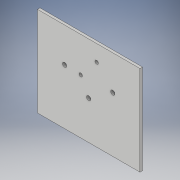
# Autodesk Inventor part: 板
Saved by Autodesk Inventor 2019 (Build 230136000, 136)
## iProperties
Created: 2020-09-25
Part Number: 板
Material: 一般
Document SubType Name: Modeling
Designer: Toshihito
Density: 1 g/cm^3
Appearance: 既定
Author: Toshihito
Autodesk Inventor part; units mm, degrees
ref_plane "YZ Plane" through (0, 0, 0) normal (1, 0, 0) x (0, 1, 0)
ref_plane "XZ Plane" through (0, 0, 0) normal (0, 1, 0) x (-1, 0, 0)
ref_plane "XY Plane" through (0, 0, 0) normal (0, 0, 1) x (1, 0, 0)
sketch "スケッチ1" plane through (0, 0, 0) normal (0, 0, 1) x (1, 0, 0)
  line L0 (-60, 52.5) -> (60, 52.5)
  line L1 (60, 52.5) -> (60, -52.5)
  line L2 (60, -52.5) -> (-60, -52.5)
  line L3 (-60, -52.5) -> (-60, 52.5)
  line L4 (-60, 52.5) -> (60, -52.5) construction
  line L5 (60, 52.5) -> (-60, -52.5) construction
  line L6 (-105.2334, 22.5) -> (96.2645, 22.5) construction
  circle A0 centre (0, -7.5) radius 2.5
  line L7 (0, 22.5) -> (28.1908, 12.2394) construction
  line L8 (0, 22.5) -> (-28.1908, 12.2394) construction
  line L9 (-9.3204, 11.3924) -> (0, 22.5) construction
  line L10 (9.3204, 33.6076) -> (0, 22.5) construction
  line L11 (0, 85.1475) -> (0, -17.897) construction
  circle A1 centre (-9.3204, 11.3924) radius 2
  circle A2 centre (9.3204, 33.6076) radius 2
  circle A3 centre (28.1908, 12.2394) radius 2.5
  circle A4 centre (-28.1908, 12.2394) radius 2.5
  point P0 (0, 0)
  dimension "d1" = 105
  dimension "d2" = 30
  dimension "d3" = 5
  dimension "d4" = 30
  dimension "d5" = 20
  dimension "d6" = 20
  dimension "d7" = 40
  dimension "d12" = 30
  dimension "d13" = 30
  dimension "d14" = 14.5
  dimension "d15" = 14.5
  dimension "d16" = 4
  dimension "d17" = 4
  dimension "d18" = 5
  dimension "d19" = 5
  constraints: 24 end point, 5 centre point, 4 coincident, 3 equal length, 2 horizontal, 2 midpoint, 2 point on line, 1 perpendicular, 1 vertical
  measures "d1" distance of L0.end L1.end
  measures "d2" distance between parallel lines of L0 L6
  measures "d3" diameter of A0
  measures "d4" distance from line of L6 A0.centre
  measures "d5" angle of L8 L6
  measures "d6" angle of L6 L7
  measures "d7" angle of L11 L10
  measures "d12" distance of L7.start L7.end
  measures "d13" distance of L7.start L8.end
  measures "d14" distance of L10.start L7.start
  measures "d15" distance of L9.start L7.start
  measures "d16" diameter of A1
  measures "d17" diameter of A2
  measures "d18" diameter of A3
  measures "d19" diameter of A4
extrude "押し出し1" add sketch "スケッチ1" along normal blind 3
